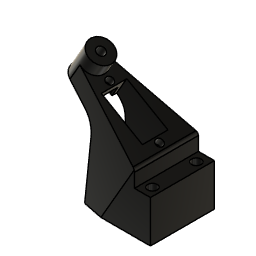
Head Tube v41 (Autodesk Fusion 360 design; units mm, degrees)
Autodesk Fusion 360 part; units mm, degrees
sketch "Main" plane through (0, 0, 0) normal (0, 1, 0) x (1, 0, 0)
  line L0 (0, 0) -> (35, 0)
  line L1 (35, 0) -> (35, -21)
  line L2 (-19.4678, -44.3397) -> (-14.4678, -53)
  line L3 (-19.4678, -44.3397) -> (0, -33.1)
  line L4 (0, -33.1) -> (0, 0)
  line L5 (-14.4678, -53) -> (27, -29.0585)
  line L6 (35, -21) -> (27, -21)
  line L7 (27, -21) -> (27, -29.0585)
  dimension "d1" = 35
  dimension "d2" = 21
  dimension "d4" = 10
  dimension "d5" = 60
  dimension "d7" = 53
  dimension "d34" = 33.1
  dimension "d35" = 8
  constraint coincident L0.start L4.end
  constraint horizontal L0
  constraint perpendicular L0 L1
  constraint perpendicular L2 L3
  constraint perpendicular L2 L5
  constraint perpendicular L1 L6
  constraint vertical L4
  constraint perpendicular L6 L7
  constraint coincident L5.end L7.end
  measures "d1" distance of L0.start L0.end
  measures "d2" distance of L0.end L1.end
  measures "d4" distance of L2.start L2.end
  measures "d5" angle of L0 L2
  measures "d7" distance of L0 L2.end
  measures "d34" distance of L3.end L0.start
  measures "d35" distance of L1.end L6.end
extrude "Extrude1" add sketch "Main" along normal blind 32
sketch "Upper Cut " plane through (19.3327, 0, 33.4853) normal (0.5, 0, 0.866025) x (0, 1, 0)
  line L0 (0, 39.0295) -> (0, -8.8534)
  line L1 (32, -8.8534) -> (32, 39.0295)
  line L2 (32, 39.0295) -> (0, 39.0295)
  line L3 (0, -30.3109) -> (32, -30.3109) construction
  line L4 (16, 39.0295) -> (16, -30.3109) construction
  arc A0 (21.8411, 34.4013) -> (10.1589, 34.4013) centre (16, 33.0295) ccw
  line L5 (10.1589, 34.4013) -> (0, -8.8534)
  line L6 (21.8411, 34.4013) -> (32, -8.8534)
  line L7 (0, -8.8534) -> (32, -8.8534)
  dimension "d11" = 6
  constraint midpoint L2 L4.start
  constraint midpoint L3 L4.end
  constraint coincident L4 A0.centre
  constraint tangent L2 A0
  constraint coincident L0.end L5.end
  constraint coincident L1.start L6.end
  constraint tangent A0 L5
  constraint coincident A0.end L5.start
  constraint tangent A0 L6
  measures "d11" radius of A0
extrude "Extrude2" cut sketch "Upper Cut " against normal blind 43 contours L0 L2 A0 L5 | L1 L2 A0 L6
sketch "Tube Extension" plane through (19.3327, 0, 33.4853) normal (0.5, 0, 0.866025) x (0, 1, 0)
  line L0 (32, -8.8534) -> (21.8411, 34.4013)
  arc A0 (21.8411, 34.4013) -> (10.1589, 34.4013) centre (16, 33.0295) ccw
  line L1 (10.1589, 34.4013) -> (0, -8.8534)
  circle A1 centre (16, 33.0295) radius 6
  line L2 (0, -8.8534) -> (32, -8.8534)
  dimension "d14" = 12
  constraint concentric A0 A1
  measures "d14" diameter of A1
extrude "Extrude3" add sketch "Tube Extension" along normal blind 7 contours A0 A1
sketch "Tube Hole" plane through (22.8327, 0, 39.5474) normal (0.5, 0, 0.866025) x (0, 1, 0)
  circle A0 centre (16, 33.0295) radius 6
  circle A1 centre (16, 33.0295) radius 2.1
  dimension "d17" = 4.2
  constraint concentric A0 A1
  measures "d17" diameter of A1
extrude "Extrude4" cut sketch "Tube Hole" against normal up to surface (17 mm away) contours A1
fillet "Fillet1" radius 10 1 edges at (0, 16, 33.1)
sketch "Servo Holes" plane through (19.3327, 0, 33.4853) normal (0.5, 0, 0.866025) x (0, 1, 0)
  arc A0 (10.1589, 34.4013) -> (21.8411, 34.4013) centre (16, 33.0295) ccw
  line L0 (10.1589, 34.4013) -> (0, -8.8534)
  line L1 (32, -8.8534) -> (21.8411, 34.4013)
  line L2 (16, 27.0295) -> (16, -8.8534) construction
  line L3 (9.6, 21.4466) -> (22.4, 21.4466)
  line L4 (22.4, 21.4466) -> (22.4, -2.3534)
  line L5 (22.4, -2.3534) -> (9.6, -2.3534)
  line L6 (9.6, -2.3534) -> (9.6, 21.4466)
  circle A1 centre (16, 23.9466) radius 1.85
  circle A2 centre (16, -4.8534) radius 1.85
  line L7 (0, -8.8534) -> (32, -8.8534)
  dimension "d22" = 12.8
  dimension "d23" = 23.8
  dimension "d24" = 6.4
  dimension "d28" = 3.7
  dimension "d29" = 3.7
  dimension "d30" = 28.8
  dimension "d31" = 2.5
  dimension "d36" = 6.5
  constraint horizontal L3
  constraint vertical L4
  constraint horizontal L5
  constraint vertical L6
  constraint coincident L2 A1.centre
  constraint coincident L2 A2.centre
  constraint midpoint L2.end L7
  constraint coincident A0 L2.start
  measures "d22" distance of L3.start L3.end
  measures "d23" distance of L3.start L5.end
  measures "d24" distance of L2 L6
  measures "d28" diameter of A1
  measures "d29" diameter of A2
  measures "d30" distance of A1.centre A2.centre
  measures "d31" distance of L5 A2.centre
  measures "d36" distance of L5 L7
extrude "Extrude5" cut sketch "Servo Holes" against normal blind 17.5 contours L3 L4 L5 L6
extrude "Extrude6" cut sketch "Servo Holes" against normal blind 4 contours A1 | A2
fillet "Fillet3" radius 2 1 edges at (27, 16, 29.0585)
sketch "Top Plate Holes" plane through (0, 0, 21) normal (0, 0, 1) x (-1, 0, 0)
  line L0 (-27, 0) -> (-35, 0)
  line L1 (-35, 0) -> (-35, -32)
  line L2 (-35, -32) -> (-27, -32)
  line L3 (-27, -32) -> (-27, 0)
  line L4 (-31, -32) -> (-31, 0) construction
  circle A0 centre (-31, -27) radius 2.4
  circle A1 centre (-31, -5) radius 2.4
  dimension "d41" = 4.8
  dimension "d42" = 4.8
  dimension "d44" = 22
  dimension "d45" = 5
  constraint midpoint L2 L4.start
  constraint midpoint L0 L4.end
  constraint coincident L4 A0.centre
  constraint coincident L4 A1.centre
  measures "d41" diameter of A0
  measures "d42" diameter of A1
  measures "d44" distance of A0.centre A1.centre
  measures "d45" distance of L0 A1.centre
extrude "Extrude7" cut sketch "Top Plate Holes" against normal blind 8 contours A0 | A1
sketch "Base Holes" plane through (0, 0, 0) normal (0, 0, -1) x (1, 0, 0)
  line L0 (10.223, 0) -> (0, -2.0793)
  line L1 (0, -2.0793) -> (0, -29.9207)
  line L2 (0, -29.9207) -> (10.223, -32)
  line L3 (10.223, -32) -> (35, -32)
  line L4 (35, -32) -> (35, 0)
  line L5 (35, 0) -> (10.223, 0)
  circle A0 centre (6, -6) radius 2.4
  circle A1 centre (29, -6) radius 2.4
  circle A2 centre (6, -26) radius 2.4
  circle A3 centre (29, -26) radius 2.4
  dimension "d59" = 4.8
  dimension "d61" = 6
  dimension "d62" = 6
  dimension "d65" = 23
  dimension "d66" = -20
  measures "d59" diameter of A0
  measures "d61" distance of L5 A0.centre
  measures "d62" distance of L1 A0.centre
extrude "Extrude8" cut sketch "Base Holes" against normal blind 8 contours A0 | A1 | A2 | A3
sketch "Servo Wires " plane through (-18.5733, 0, 10.7233) normal (0.866025, 0, -0.5) x (0, 1, 0)
  line L0 (9.6, 28.6269) -> (22.4, 28.6269)
  line L1 (22.4, 28.6269) -> (22.4, 38.6654)
  line L2 (22.4, 38.6654) -> (9.6, 38.6654)
  line L3 (9.6, 38.6654) -> (9.6, 28.6269)
  line L4 (12, 33.6269) -> (20, 33.6269)
  line L5 (20, 33.6269) -> (20, 28.6269)
  line L6 (20, 28.6269) -> (12, 28.6269)
  line L7 (12, 28.6269) -> (12, 33.6269)
  dimension "d93" = 8
  dimension "d94" = 2.4
  dimension "d95" = 5
  constraint horizontal L4
  constraint vertical L5
  constraint horizontal L6
  constraint vertical L7
  constraint coincident L0 L5.end
  measures "d93" distance of L4.start L4.end
  measures "d94" distance of L3 L7
  measures "d95" distance of L4.end L5.end
extrude "Extrude9" cut sketch "Servo Wires " against normal blind 2 contours L0 L4 L5 L6 L7
fillet "Fillet4" radius 1 3 edges at (-1.7598, 16, 39.8451) (-4.7323, 12, 38.6967) (-4.7323, 20, 38.6967)
